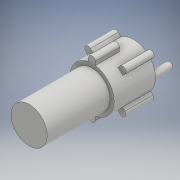
# Autodesk Inventor part: Pompe
Saved by Autodesk Inventor 2018 (Build 220112000, 112)
## iProperties
Created: 2018-04-06
Part Number: Pompe
Material: Générique
Document SubType Name: Modeling
Designer: Dimitri
Density: 1 g/cm^3
Appearance: Par défaut
Author: Dimitri
Autodesk Inventor part; units mm, degrees
ref_plane "YZ Plane" through (0, 0, 0) normal (1, 0, 0) x (0, 1, 0)
ref_plane "XZ Plane" through (0, 0, 0) normal (0, 1, 0) x (-1, 0, 0)
ref_plane "XY Plane" through (0, 0, 0) normal (0, 0, 1) x (1, 0, 0)
sketch "Esquisse1" plane through (0, 0, 0) normal (0, 1, 0) x (-1, 0, 0)
  circle A0 centre (0, 0) radius 13.5
  dimension "d0" = 27
  constraints: 1 centre point, 1 coincident
  measures "d0" diameter of A0
extrude "Extrusion1" add sketch "Esquisse1" along normal blind 47
sketch "Esquisse2" plane through (0, 47, 0) normal (0, 1, 0) x (1, 0, 0)
  circle A0 centre (0, 0) radius 16.5
  arc A1 (2.5, 19) -> (-2.5, 19) centre (0, 19) ccw
  line L0 (2.5, -19) -> (2.5, -16.3095)
  line L1 (2.5, 19) -> (2.5, 16.3095)
  line L2 (-2.5, 19) -> (-2.5, 16.3095)
  line L3 (-2.5, -19) -> (-2.5, -16.3095)
  arc A2 (-2.5, -19) -> (2.5, -19) centre (0, -19) ccw
  dimension "d3" = 33
  dimension "d4" = 5
  dimension "d7" = 19
  constraints: 8 end point, 8 point on circle, 3 centre point, 2 point on line, 2 tangent, 1 coincident, 1 vertical
  measures "d3" diameter of A0
  measures "d4" diameter of A1
  measures "d7" distance of A0.centre A1.centre
extrude "Extrusion2" add sketch "Esquisse2" along normal blind 10
sketch "Esquisse3" plane through (0, 57, 0) normal (0, 1, 0) x (1, 0, 0)
  arc A0 (2.5, 19) -> (-2.5, 19) centre (0, 19) ccw
  line L0 (-2.5, 19) -> (-2.5, 16.3095)
  line L1 (2.5, 16.3095) -> (2.5, 19) projected
  line L2 (2.5, 19) -> (2.5, 16.3095)
  arc A1 (-2.5, -19) -> (2.5, -19) centre (0, -19) ccw
  line L3 (-2.5, -19) -> (-2.5, -16.3095)
  line L4 (2.5, -16.3095) -> (2.5, -19)
  arc A2 (-11.1964, 15.5528) -> (-14.8385, 12.1272) centre (-13.0175, 13.84) ccw
  line L5 (-11.1964, 15.5528) -> (-9.3531, 13.593)
  line L6 (-14.8385, 12.1272) -> (-12.9952, 10.1674)
  arc A3 (-14.8385, -12.1272) -> (-11.1964, -15.5528) centre (-13.0175, -13.84) ccw
  line L7 (-11.1964, -15.5528) -> (-9.3531, -13.593)
  line L8 (-14.8385, -12.1272) -> (-12.9952, -10.1674)
  arc A4 (14.5441, 12.2779) -> (10.8671, 15.666) centre (12.7056, 13.9719) ccw
  line L9 (10.8671, 15.666) -> (9.1089, 13.7578)
  line L10 (14.5441, 12.2779) -> (12.8117, 10.3976)
  line L11 (11.1741, -15.4495) -> (9.3774, -13.5763)
  arc A5 (11.1741, -15.4495) -> (14.7929, -11.9752) centre (12.9835, -13.7124) ccw
  line L12 (14.7929, -11.9752) -> (13.023, -10.1317)
  arc A6 (13.023, -10.1317) -> (12.8117, 10.3976) centre (0, 0) ccw
  arc A7 (-12.9952, 10.1674) -> (-13.1739, 9.9347) centre (0, 0) ccw
  arc A8 (9.1089, 13.7578) -> (2.5, 16.3095) centre (0, 0) ccw
  arc A9 (9.1089, 13.7578) -> (2.5, 16.3095) centre (0, 0) ccw
  arc A10 (-2.5, 16.3095) -> (-2.5, -16.3095) centre (0, 0) ccw projected
  arc A11 (-2.5, 16.3095) -> (-9.3531, 13.593) centre (0, 0) ccw
  arc A12 (-12.9952, 10.1674) -> (-12.9952, -10.1674) centre (0, 0) ccw
  arc A13 (-9.3531, -13.593) -> (-2.5, -16.3095) centre (0, 0) ccw
  line L13 (2.5, -19) -> (2.5, -16.3095) projected
  arc A14 (2.5, -16.3095) -> (9.3774, -13.5763) centre (0, 0) ccw
  arc A15 (13.023, -10.1317) -> (12.8117, 10.3976) centre (0, 0) ccw
  constraints: 32 point on circle, 24 end point, 15 centre point, 8 coincident, 2 equal length, 2 tangent, 1 point on line
extrude "Extrusion3" add sketch "Esquisse3" along normal blind 8
sketch "Esquisse5" plane through (0, 65, 0) normal (0, 1, 0) x (1, 0, 0)
  arc A0 (9.1089, 13.7578) -> (2.5, 16.3095) centre (0, 0) ccw projected
  arc A1 (-2.5, 16.3095) -> (-9.3531, 13.593) centre (0, 0) ccw projected
  line L0 (-9.3531, 13.593) -> (-11.1964, 15.5528) projected
  arc A2 (-11.1964, 15.5528) -> (-14.8385, 12.1272) centre (-13.0175, 13.84) ccw projected
  line L1 (-14.8385, 12.1272) -> (-12.9952, 10.1674) projected
  arc A3 (-12.9952, 10.1674) -> (-12.9952, -10.1674) centre (0, 0) ccw projected
  line L2 (-12.9952, -10.1674) -> (-14.8385, -12.1272) projected
  arc A4 (-14.8385, -12.1272) -> (-11.1964, -15.5528) centre (-13.0175, -13.84) ccw projected
  line L3 (-11.1964, -15.5528) -> (-9.3531, -13.593) projected
  arc A5 (-9.3531, -13.593) -> (-2.5, -16.3095) centre (0, 0) ccw projected
  arc A6 (2.5, -16.3095) -> (9.3774, -13.5763) centre (0, 0) ccw projected
  line L4 (9.3774, -13.5763) -> (11.1741, -15.4495) projected
  arc A7 (11.1741, -15.4495) -> (14.7929, -11.9752) centre (12.9835, -13.7124) ccw projected
  line L5 (14.7929, -11.9752) -> (13.023, -10.1317) projected
  arc A8 (13.023, -10.1317) -> (12.8117, 10.3976) centre (0, 0) ccw projected
  arc A9 (14.5441, 12.2779) -> (10.8671, 15.666) centre (12.7056, 13.9719) ccw projected
  line L6 (10.8671, 15.666) -> (9.1089, 13.7578) projected
  line L7 (12.8117, 10.3976) -> (14.5441, 12.2779) projected
  arc A10 (2.5, 16.3095) -> (-2.5, 16.3095) centre (0, 0) ccw
  arc A11 (-2.5, -16.3095) -> (2.5, -16.3095) centre (0, 0) ccw
  constraints: 4 point on circle, 2 centre point, 2 coincident
extrude "Extrusion4" add sketch "Esquisse5" along normal blind 13
sketch "Esquisse6" plane through (0, 78, 0) normal (0, 1, 0) x (1, 0, 0)
  circle A0 centre (14, 0) radius 2.5
  circle A1 centre (-8, 0) radius 2.5
  point P0 (0, 0)
  point P1 (0, 0)
  dimension "d20" = 5
  dimension "d21" = 5
  dimension "d24" = 8
  constraints: 2 centre point
  measures "d20" diameter of A0
  measures "d21" diameter of A1
  measures "d24" distance of point (0, 0) A1.centre
extrude "Extrusion5" add sketch "Esquisse6" along normal blind 13
shell "Coque1" thickness 0.5 removed faces 2 at (-7.4475, 91, 0.0341) at (13.3413, 91, 0.3326)
